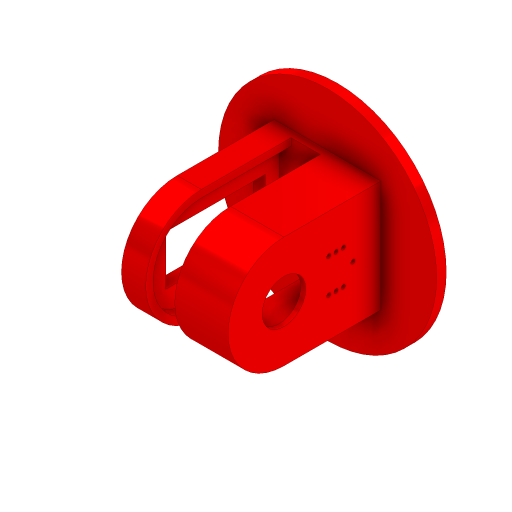
# Autodesk Inventor part: arm_base
Saved by Autodesk Inventor 2023 (Build 270158000, 158)
## iProperties
Created: 2023-01-08
Part Number: arm_base
Material: PLA plastic
Document SubType Name: Modeling
Designer: denyh
Density: 1.25 g/cm^3
Appearance: Generic
Author: denyh
Autodesk Inventor part; units mm, degrees
ref_plane "YZ Plane" through (0, 0, 0) normal (1, 0, 0) x (0, 1, 0)
ref_plane "XZ Plane" through (0, 0, 0) normal (0, 1, 0) x (-1, 0, 0)
ref_plane "XY Plane" through (0, 0, 0) normal (0, 0, 1) x (1, 0, 0)
sketch "Sketch1" plane through (0, 0, 0) normal (0, 0, 1) x (1, 0, 0)
  circle A0 centre (0, 0) radius 45
  dimension "d0" = 90
  constraints: 1 centre point, 1 coincident
  measures "d0" diameter of A0
extrude "Extrusion1" add sketch "Sketch1" along normal blind 4
sketch "Sketch4" plane through (0, 0, 0) normal (1, 0, 0) x (0, 1, 0)
  line L0 (45, 4) -> (-45, 4) projected
  line L1 (45, 4) -> (35, 4)
  line L2 (35, 4) -> (35, 67)
  line L3 (-45, 4) -> (-35, 4)
  line L4 (0, 0) -> (0, 79.3113)
  line L5 (0, 64) -> (0, 44)
  circle A0 centre (0, 44) radius 23
  circle A1 centre (0, 44) radius 20
  circle A2 centre (0, 44) radius 9
  line L6 (0, 44) -> (10.25, 44) construction
  line L7 (35, 67) -> (-35, 67)
  line L8 (-35, 67) -> (-35, 4)
  line L9 (0, 44) -> (0, 54.25)
  line L10 (0, 44) -> (-10.25, 44)
  line L11 (-10.25, 44) -> (-10.25, 53.7227)
  line L12 (-10.25, 53.7227) -> (10.25, 53.7227)
  line L13 (10.25, 53.7227) -> (10.25, 12.7227)
  line L14 (10.25, 12.7227) -> (-10.25, 12.7227)
  line L15 (-10.25, 12.7227) -> (-10.25, 53.7227)
  dimension "d12" = 10
  dimension "d13" = 63
  dimension "d14" = 10
  dimension "d15" = 20
  dimension "d16" = 46
  dimension "d17" = 40
  dimension "d18" = 18
  dimension "d94" = 10.25
  dimension "d95" = 10.25
  dimension "d96" = 41
  dimension "d97" = 20.5
  constraints: 30 end point, 6 point on line, 4 perpendicular, 3 centre point, 3 coincident, 3 horizontal, 2 vertical, 1 parallel
  measures "d12" distance of L0.start L1.end
  measures "d13" distance of L1.end L2.end
  measures "d14" distance of L0.end L3.end
  measures "d15" distance of L5.start L5.end
  measures "d16" diameter of A0
  measures "d17" diameter of A1
  measures "d18" diameter of A2
  measures "d94" distance of L9.start L9.end
  measures "d95" distance of L9.start L10.end
  measures "d96" distance of L12.end L13.end
  measures "d97" distance of L13.end L14.end
sketch "Sketch7" plane through (0, 0, 0) normal (1, 0, 0) x (0, 1, 0)
  circle A0 centre (0, 44) radius 23 projected
  line L0 (23, 44) -> (23, 4)
  line L1 (45, 4) -> (-45, 4) projected
  line L2 (23, 4) -> (-45, 4)
  line L3 (0, 44) -> (-18.4261, 62.4261)
  line L4 (0, 44) -> (26.0584, 44) construction
  line L5 (-23, 44) -> (-23, 4)
  line L6 (23, 4) -> (-23, 4)
  point P0 (0, 0)
  point P1 (-16.2635, 60.2635)
  point P2 (-23, 4)
  dimension "d32" = 135
  constraints: 12 end point, 3 point on circle, 3 point on line, 2 horizontal, 1 collinear, 1 equal length, 1 perpendicular, 1 tangent, 1 vertical
  measures "d32" angle of L4 L3
extrude "Extrusion4" add sketch "Sketch7" along normal blind 20
sketch "Sketch9" plane through (0, 0, 0) normal (-1, 0, 0) x (0, 0, 1)
  circle A0 centre (44, 0) radius 20 projected
  arc A1 (44, -23) -> (44, 23) centre (44, 0) ccw projected
  line L0 (44, 20) -> (4, 20)
  line L1 (4, 0) -> (4, 45) projected
  line L2 (4, 23) -> (44, 23) projected
  line L3 (4, -45) -> (4, -42)
  line L4 (44, -20) -> (4, -20)
  line L5 (4, -20) -> (4, 20)
  point P0 (0, 0)
  dimension "d37" = 3
  constraints: 8 end point, 2 horizontal, 2 point on circle, 2 point on line, 1 collinear, 1 tangent
  measures "d37" distance of L3.start L3.end
extrude "Extrusion6" cut sketch "Sketch9" against normal blind 7
extrude "Extrusion7" cut sketch "Sketch4" along normal blind 19 contours L14 L15 A0 L4 | L4 A0 L13 L14 | A0 L15 A1 L4 | L4 A1 L13 A0 | A1 L15 L10 A2 L4 | L4 A2 L12 L13 A1 | A2 L10 L4 | L4 A2 | L4 A2 L10 L11 L12 | L10 A2 L4 picked at (-9.1739, 25.1699) picked at (9.1739, 25.1699)
extrude "Extrusion8" cut sketch "Sketch4" along normal blind 20 contours A2 L10 L4 | L4 A2 | L10 A2 L4
sketch "Sketch15" plane through (19, 0, 0) normal (-1, 0, 0) x (0, 0, 1)
  line L0 (51.2478, 7.2478) -> (91.2478, 7.2478) construction
  line L1 (12.7227, -10.25) -> (12.7227, 10.25) projected
  line L2 (12.7227, 0) -> (15.5227, 0)
  circle A0 centre (15.5227, 0) radius 0.85
  line L3 (12.7227, 0) -> (19.5227, 0)
  circle A1 centre (19.5227, 7) radius 0.85
  circle A2 centre (22.5227, 7) radius 0.85
  circle A3 centre (25.5227, 7) radius 0.85
  line L4 (12.7227, 0) -> (26.0036, 0)
  circle A4 centre (19.5227, -7) radius 0.85
  circle A5 centre (22.5227, -7) radius 0.85
  circle A6 centre (25.5227, -7) radius 0.85
  point P0 (0, 0)
  dimension "d98" = 2.8
  dimension "d99" = 1.7
  dimension "d100" = 6.8
  dimension "d102" = 1.7
  dimension "d105" = 1.7
  dimension "d106" = 1.7
  constraints: 8 end point, 7 centre point, 3 horizontal, 3 symmetric about line, 1 coincident, 1 midpoint, 1 point on line, 3 other
  measures "d98" distance of L2.start L2.end
  measures "d99" diameter of A0
  measures "d100" distance of L2.start L3.end
  measures "d102" diameter of A1
  measures "d105" diameter of A2
  measures "d106" diameter of A3
extrude "Extrusion13" cut sketch "Sketch15" against normal blind 5
sketch "Sketch23" plane through (0, 0, 4) normal (0, 0, 1) x (1, 0, 0)
  line L0 (0, 20) -> (0, -20) projected
  line L1 (0, 23) -> (-20, 23)
  line L2 (-20, 23) -> (-20, -23)
  line L3 (-20, -23) -> (0, -23)
  line L4 (7, 20) -> (7, 23)
  line L5 (0, 23) -> (20, 23) projected
  line L6 (7, 23) -> (0, 23)
  line L7 (7, 20) -> (7, -23)
  line L8 (20, -23) -> (0, -23) projected
  point P0 (0, 0)
  point P1 (0, 26)
  point P2 (23, -23)
  dimension "d107" = 20
  constraints: 12 end point, 2 perpendicular, 2 point on line, 2 vertical, 1 collinear, 1 horizontal
  measures "d107" distance of L1.start L1.end
extrude "Extrusion21" add sketch "Sketch23" along normal blind 3
sketch "Sketch11" plane through (0, 0, 0) normal (0, 0, -1) x (-1, 0, 0)
  circle A0 centre (0, 0) radius 45 projected
  circle A1 centre (0, 0) radius 45 projected
  line L0 (0, 0) -> (0, 7.25)
  line L1 (0, 23) -> (0, -16.2635) projected
  line L2 (0, 7.25) -> (0, -7.25)
  circle A2 centre (0, 7.25) radius 1.5
  circle A3 centre (0, -7.25) radius 1.5
  point P0 (0, 10.25)
  point P1 (0, -10.25)
  point P2 (0, -23)
  dimension "d47" = 7.25
  dimension "d48" = 14.5
  dimension "d49" = 3
  dimension "d50" = 3
  constraints: 4 end point, 2 centre point, 2 coincident, 2 point on line
  measures "d47" distance of L0.start L0.end
  measures "d48" distance of L0.end L2.end
  measures "d49" diameter of A2
  measures "d50" diameter of A3
extrude "Extrusion10" cut sketch "Sketch11" along normal mid plane 20 contours A2 L1 L0 | L0 L1 A2 | A3 L1 | L1 A3
sketch "Sketch24" plane through (0, 0, 7) normal (0, 0, 1) x (1, 0, 0)
  circle A0 centre (0, 7.25) radius 1.5 projected
  circle A1 centre (0, 7.25) radius 4
  circle A2 centre (0, -7.25) radius 1.5 projected
  circle A3 centre (0, -7.25) radius 4
  point P0 (0, 0)
  dimension "d110" = 8
  dimension "d111" = 8
  constraints: 2 centre point, 2 coincident
  measures "d110" diameter of A1
  measures "d111" diameter of A3
extrude "Extrusion22" cut sketch "Sketch24" against normal blind 3
sketch "Sketch25" plane through (-20, -23, 4) normal (-1, 0, 0) x (0, 0, 1)
  arc A0 (40, 0) -> (40, 46) centre (40, 23) ccw projected
  line L0 (3, 46) -> (40, 46) projected
  line L1 (40, 0) -> (3, 0) projected
  line L2 (0, 46) -> (3, 46) projected
  line L3 (0, 46) -> (0, 0)
  line L4 (0, 0) -> (3, 0) projected
  line L5 (3, 0) -> (0, 0)
  point P0 (-4, 23)
  constraints: 4 end point, 1 vertical
extrude "Extrusion23" add sketch "Sketch25" against normal blind 8
sketch "Sketch26" plane through (-12, -23, 4) normal (1, 0, 0) x (0, 0, -1)
  arc A0 (-40, 43) -> (-40, 3) centre (-40, 23) ccw projected
  line L0 (-40, 3) -> (-3, 3) projected
  line L1 (-3, 43) -> (-40, 43) projected
  line L2 (-3, 46) -> (-3, 0) projected
  point P0 (4, 23)
extrude "Extrusion24" cut sketch "Sketch26" against normal blind 5
sketch "Sketch27" plane through (-20, -23, 4) normal (-1, 0, 0) x (0, 0, 1)
  line L0 (8.7227, 33.25) -> (49.7227, 33.25) projected
  line L1 (49.7227, 33.25) -> (49.7227, 12.75) projected
  line L2 (49.7227, 12.75) -> (8.7227, 12.75) projected
  line L3 (8.7227, 12.75) -> (8.7227, 33.25) projected
  point P0 (-4, 23)
extrude "Extrusion25" cut sketch "Sketch27" against normal blind 5
sketch "Sketch29" plane through (0, 0, 0) normal (0, 0, -1) x (-1, 0, 0)
  circle A0 centre (0, 0) radius 11
  dimension "d125" = 22
  constraints: 1 centre point, 1 coincident
  measures "d125" diameter of A0
extrude "Extrusion26" cut sketch "Sketch29" against normal blind 1.5
sketch "Sketch32" plane through (20, 0, 0) normal (1, 0, 0) x (0, 0, -1)
  circle A0 centre (-19.5227, 7) radius 0.85 projected
  circle A1 centre (-19.5227, -7) radius 0.85 projected
  circle A2 centre (-15.5227, 0) radius 0.85 projected
  circle A3 centre (-22.5227, 7) radius 0.85 projected
  circle A4 centre (-25.5227, -7) radius 0.85 projected
  circle A5 centre (-22.5227, -7) radius 0.85 projected
  circle A6 centre (-25.5227, 7) radius 0.85 projected
  circle A7 centre (-44, 0) radius 9 projected
  arc A8 (-44, 23) -> (-44, -23) centre (-44, 0) ccw projected
  line L0 (-44, -23) -> (-4, -23) projected
  line L1 (-4, 23) -> (-4, -23) projected
  line L2 (-4, 23) -> (-44, 23) projected
  point P0 (0, 0)
extrude "Extrusion27" add sketch "Sketch32" along normal blind 1
sketch "Sketch33" plane through (-20, -23, 4) normal (-1, 0, 0) x (0, 0, 1)
  line L0 (49.7227, 33.25) -> (49.7227, 12.75) projected
  line L1 (49.7227, 12.75) -> (8.7227, 12.75) projected
  line L2 (8.7227, 12.75) -> (8.7227, 33.25) projected
  line L3 (8.7227, 33.25) -> (49.7227, 33.25) projected
  line L4 (0, 0) -> (0, 46) projected
  line L5 (0, 0) -> (40, 0) projected
  arc A0 (40, 0) -> (40, 46) centre (40, 23) ccw projected
  line L6 (0, 46) -> (40, 46) projected
  point P0 (-4, 23)
extrude "Extrusion28" add sketch "Sketch33" along normal blind 1
sketch "Sketch34" plane through (19, 0, 0) normal (-1, 0, 0) x (0, 0, 1)
  circle A0 centre (19.5227, 7) radius 0.85 projected
  circle A1 centre (19.5227, -7) radius 0.85 projected
  circle A2 centre (15.5227, 0) radius 0.85 projected
  circle A3 centre (22.5227, 7) radius 0.85 projected
  circle A4 centre (25.5227, -7) radius 0.85 projected
  circle A5 centre (22.5227, -7) radius 0.85 projected
  circle A6 centre (25.5227, 7) radius 0.85 projected
  circle A7 centre (44, 0) radius 9 projected
  line L0 (53.7227, -10.25) -> (12.7227, -10.25) projected
  line L1 (53.7227, 10.25) -> (53.7227, -10.25) projected
  line L2 (12.7227, 10.25) -> (53.7227, 10.25) projected
  line L3 (12.7227, -10.25) -> (12.7227, 10.25) projected
  point P0 (0, 0)
extrude "Extrusion29" cut sketch "Sketch34" against normal blind 1
sketch "Sketch36" plane through (21, 0, 0) normal (1, 0, 0) x (0, 0, -1)
  line L0 (-7, 20) -> (-44, 20) projected
  arc A0 (-44, 23) -> (-44, -23) centre (-44, 0) ccw projected
  line L1 (-44, -23) -> (-4, -23) projected
  line L2 (-4, 23) -> (-4, -23) projected
  line L3 (-4, 23) -> (-44, 23) projected
  circle A1 centre (-19.5227, 7) radius 0.85 projected
  circle A2 centre (-19.5227, -7) radius 0.85 projected
  circle A3 centre (-15.5227, 0) radius 0.85 projected
  circle A4 centre (-22.5227, 7) radius 0.85 projected
  circle A5 centre (-25.5227, -7) radius 0.85 projected
  circle A6 centre (-22.5227, -7) radius 0.85 projected
  circle A7 centre (-25.5227, 7) radius 0.85 projected
  circle A8 centre (-44, 0) radius 9 projected
  point P0 (0, 0)
extrude "Extrusion30" add sketch "Sketch36" along normal blind 1
sketch "Sketch37" plane through (-21, -23, 4) normal (-1, 0, 0) x (0, 0, 1)
  line L0 (40, 46) -> (0, 46) projected
  line L1 (0, 0) -> (0, 46) projected
  line L2 (0, 0) -> (40, 0) projected
  arc A0 (40, 0) -> (40, 46) centre (40, 23) ccw projected
  line L3 (49.7227, 33.25) -> (49.7227, 12.75) projected
  line L4 (49.7227, 12.75) -> (8.7227, 12.75) projected
  line L5 (8.7227, 12.75) -> (8.7227, 33.25) projected
  line L6 (8.7227, 33.25) -> (49.7227, 33.25) projected
  point P0 (-4, 23)
extrude "Extrusion31" add sketch "Sketch37" along normal blind 1
body "Solid1"
